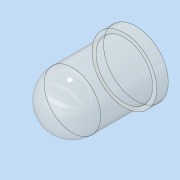
# Autodesk Inventor part: 5mmLED
Saved by Autodesk Inventor 2017 (Build 210142000, 142)
## iProperties
Created: 2016-12-16
Part Number: 5mmLED
Material: PBT Plastic
Document SubType Name: Modeling
Designer: techn
Density: 1.31 g/cm^3
Appearance: Clear
Author: techn
Autodesk Inventor part; units mm, degrees
ref_plane "YZ Plane" through (0, 0, 0) normal (1, 0, 0) x (0, 1, 0)
ref_plane "XZ Plane" through (0, 0, 0) normal (0, 1, 0) x (-1, 0, 0)
ref_plane "XY Plane" through (0, 0, 0) normal (0, 0, 1) x (1, 0, 0)
sketch "Sketch1" plane through (0, 0, 0) normal (0, 1, 0) x (-1, 0, 0)
  line L0 (0, 0) -> (2.8, 0)
  arc A0 (2.45, 5.5) -> (0, 7.95) centre (0, 5.5) ccw
  line L1 (0, 7.95) -> (0, 0)
  line L2 (2.8, 0) -> (2.8, 1)
  line L3 (0, 1) -> (2.45, 1)
  line L4 (2.45, 1) -> (2.45, 5.5)
  line L5 (2.45, 1) -> (2.8, 1)
  dimension "d0" = 2.8
  dimension "d2" = 1
  dimension "d3" = 2.45
  dimension "d4" = 5.5
  constraints: 12 end point, 2 horizontal, 2 perpendicular, 2 point on circle, 2 vertical, 1 centre point, 1 line through centre, 1 point on line, 1 tangent
  measures "d0" distance of L0.start L0.end
  measures "d2" distance of L0.end L2.end
  measures "d3" distance of L3.start L3.end
  measures "d4" distance from line of L4.end L0
revolve "Revolution1" add sketch "Sketch1" angle 360 about axis through (0, 0, 7.95) along (0, 0, -1)
body "Solid1"
